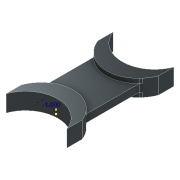
# Autodesk Inventor part: dc motor holder 2
Saved by Autodesk Inventor 2021 (Build 250183000, 183)
## iProperties
Created: 2021-06-22
Part Number: dc motor holder 2
Material: Iron, Ductile
Document SubType Name: Modeling
Designer: user
Density: 7.15 g/cm^3
Appearance: Iron Gray
Author: user
Autodesk Inventor part; units mm, degrees
ref_plane "YZ Plane" through (0, 0, 0) normal (1, 0, 0) x (0, 1, 0)
ref_plane "XZ Plane" through (0, 0, 0) normal (0, 1, 0) x (-1, 0, 0)
ref_plane "XY Plane" through (0, 0, 0) normal (0, 0, 1) x (1, 0, 0)
sketch "Sketch1" plane through (0, 0, 0) normal (0, 1, 0) x (-1, 0, 0)
  point P0 (0, 0)
sketch "Sketch2" plane through (0, 0, 0) normal (0, 1, 0) x (-1, 0, 0)
  line L0 (0, 0) -> (38.1, 0)
  line L1 (38.1, 0) -> (38.1, -84.0465)
  arc A0 (50.8, -121.2155) -> (0, -85.725) centre (0, -139.827) ccw
  line L2 (38.1, -84.0465) -> (38.1, -101.4159)
  arc A1 (50.8, -146.6155) -> (0, -111.125) centre (0, -165.227) ccw
  line L3 (50.8, -121.2155) -> (50.8, -146.6155)
  line L4 (0, 0) -> (0, -111.125)
  constraints: 10 end point, 5 point on circle, 4 vertical, 2 centre point, 1 coincident, 1 horizontal, 1 point on line
sketch "Sketch3" plane through (0, 0, 0) normal (0, 1, 0) x (-1, 0, 0)
  point P0 (0, 0)
  point P1 (0, 0)
  point P2 (16.5768, 0)
  point P3 (25.4, 0)
  point P4 (0, 0)
  dimension "d10" = 25.4
  constraints: 2 coincident
  measures "d10" distance of point (0, 0) point (25.4, 0)
extrude "Extrusion1" add sketch "Sketch2" along normal blind 6.35
sketch "Sketch4" plane through (0, 6.35, 0) normal (0, 1, 0) x (1, 0, 0)
  arc A0 (-50.8, 121.2155) -> (-38.1, 101.4159) centre (0, 139.827) ccw projected
  arc A1 (-50.8, 146.6155) -> (0, 111.125) centre (0, 165.227) ccw projected
  line L0 (-50.8, 146.6155) -> (-50.8, 121.2155) projected
  line L1 (-50.8, 121.2155) -> (-50.8, 146.6155)
  line L2 (0, 111.125) -> (0, 92.3126)
  line L3 (0, 0) -> (0, 111.125) projected
  arc A2 (-42.5277, 131.7842) -> (0, 111.125) centre (0, 165.227) ccw
  arc A3 (-50.8, 121.2155) -> (0, 92.3126) centre (-9.952, 133.9155) ccw
  arc A4 (-50.8, 146.6155) -> (-44.1205, 133.9155) centre (0, 165.227) ccw
  arc A5 (-50.8, 146.6155) -> (0, 111.125) centre (0, 165.227) ccw
  point P0 (-40.6454, 104.1202)
  constraints: 12 point on circle, 4 centre point, 4 end point, 2 coincident, 2 concentric, 2 point on line, 1 vertical
extrude "Extrusion2" add sketch "Sketch4" along normal blind 7.62 contours L0 A1 L2 A3 A0
mirror "Mirror1" about plane through (0, 0, 0) normal (1, 0, 0) of "Extrusion1", "Extrusion2"
sketch "Sketch5" plane through (0, 6.35, 0) normal (0, 1, 0) x (1, 0, 0)
  arc A0 (38.1, 101.4159) -> (50.8, 121.2155) centre (0, 139.827) ccw projected
  arc A1 (-38.1, 101.4159) -> (38.1, 101.4159) centre (0, 137.2023) ccw
  line L0 (-38.1, 101.4159) -> (-38.1, 0) projected
  arc A2 (-38.1, 101.4159) -> (38.1, 101.4159) centre (0, 209.31) ccw
  point P0 (0, 0)
  constraints: 4 point on circle, 2 centre point
extrude "Extrusion3" add sketch "Sketch5" along normal blind 7.62
mirror "Mirror2" about plane through (0, 0, 0) normal (0, 1, 0) of "Extrusion1", "Extrusion2", "Mirror1", "Extrusion3"
sketch "Sketch6" plane through (0, 6.35, 0) normal (0, 1, 0) x (1, 0, 0)
  line L0 (-38.1, 101.4159) -> (-38.1, 0) projected
  line L1 (38.1, 101.4159) -> (38.1, 0) projected
  line L2 (-38.1, -38.1) -> (38.1, -38.1)
  line L3 (38.1, -38.1) -> (38.1, 38.1)
  line L4 (38.1, 38.1) -> (-38.1, 38.1)
  line L5 (-38.1, 38.1) -> (-38.1, -38.1)
  point P0 (0, 0)
  point P1 (-38.1, -101.4159)
  point P2 (-38.1, 38.1)
  point P3 (38.1, -101.4159)
  point P4 (-38.1, 0)
  dimension "d17" = 38.1
  dimension "d18" = 38.1
  constraints: 9 end point, 3 point on line, 2 parallel, 1 horizontal, 1 perpendicular
  measures "d17" distance of L0.end L2.start
  measures "d18" distance of point (-38.1, 38.1) L0.end
extrude "Extrusion4" cut sketch "Sketch6" against normal through all
sketch "Sketch7" plane through (0, -6.35, -137.2023) normal (0, -1, 0) x (1, 0, 0)
  point P0 (0, 137.2023)
sketch "Sketch8" plane through (-38.1, 6.35, -38.1) normal (0, 0, 1) x (1, 0, 0)
  line L0 (0, 0) -> (76.2, 0) projected
  line L1 (76.2, -12.7) -> (76.2, -20.32) projected
  line L2 (0, 0) -> (76.2, 0)
  line L3 (76.2, 0) -> (76.2, -12.7)
  line L4 (76.2, -12.7) -> (0, -12.7)
  line L5 (0, -12.7) -> (0, 0)
  point P0 (38.1, -6.35)
  constraints: 8 end point, 2 parallel, 1 horizontal, 1 perpendicular
extrude "Extrusion5" cut sketch "Sketch8" against normal blind 12.7
sketch "Sketch9" plane through (-38.1, 6.35, -50.8) normal (0, 0, 1) x (1, 0, 0)
  line L0 (0, 0) -> (76.2, 0) projected
  line L1 (76.2, 0) -> (76.2, -12.7) projected
  line L2 (0, 0) -> (76.2, 0)
  line L3 (76.2, 0) -> (76.2, -12.7)
  line L4 (76.2, -12.7) -> (0, -12.7)
  line L5 (0, -12.7) -> (0, 0)
  point P0 (38.1, -6.35)
  constraints: 8 end point, 2 parallel, 1 horizontal, 1 perpendicular
extrude "Extrusion6" cut sketch "Sketch9" against normal blind 25.4
sketch "Sketch10" plane through (38.1, -6.35, -101.4159) normal (1, 0, 0) x (0, 0, -1)
  point P0 (-101.4159, 6.35)
sketch "Sketch11" plane through (-38.1, 6.35, -76.2) normal (0, 0, 1) x (1, 0, 0)
  line L0 (0, -12.7) -> (-2.5454, -12.7) projected
  line L1 (76.2, 0) -> (76.2, -12.7) projected
  line L2 (0, -12.7) -> (76.2, -12.7)
  line L3 (76.2, -12.7) -> (76.2, 0)
  line L4 (76.2, 0) -> (0, 0)
  line L5 (0, 0) -> (0, -12.7)
  point P0 (38.1, -6.35)
  constraints: 8 end point, 2 parallel, 1 horizontal, 1 perpendicular
extrude "Extrusion7" add sketch "Sketch11" along normal blind 19.05
mirror "Mirror4" about plane through (0, 0, -57.15) normal (0, 0, 1)
body "Solid1"
